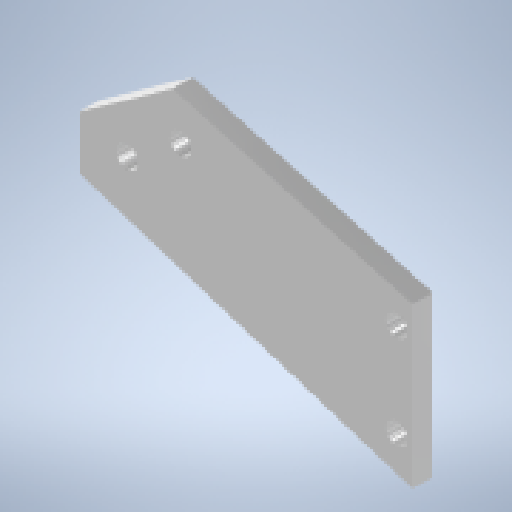
# Autodesk Inventor part: antana_side
Saved by Autodesk Inventor 2024.1 (Build 281209000, 209)
## iProperties
Created: 2024-02-25
Part Number: antana_side
Material: アルミニウム 6061
Document SubType Name: Sheet Metal
Designer: hibik
Density: 2.7 g/cm^3
Sheet Metal Rule: Default_mm
Appearance: アルミニウム - フラット
Author: hibik
Autodesk Inventor part; units mm, degrees
ref_plane "YZ Plane" through (0, 0, 0) normal (1, 0, 0) x (0, 1, 0)
ref_plane "XZ Plane" through (0, 0, 0) normal (0, 1, 0) x (-1, 0, 0)
ref_plane "XY Plane" through (0, 0, 0) normal (0, 0, 1) x (1, 0, 0)
sketch "スケッチ1" plane through (0, 0, 0) normal (0, 0, 1) x (1, 0, 0)
  line L0 (-25, 8) -> (-25, 12)
  line L1 (-25, 12) -> (0, 12)
  line L2 (0, 12) -> (0, 0)
  line L3 (0, 0) -> (-25, 8)
  line L4 (0, 12) -> (-18, 17)
  line L5 (-18, 17) -> (-25, 12)
  dimension "d0" = 12
  dimension "d2" = 4
  dimension "d4" = 25
  dimension "d7" = 5
  dimension "d8" = 18
  measures "d0" distance of L1.end L2.end
  measures "d2" distance of L0.start L0.end
  measures "d4" distance between parallel lines of L2 L0
  measures "d7" distance from line of L1 L4.end
  measures "d8" distance from line of L2 L4.end
extrude "プレート1" add sketch "スケッチ1" along normal blind 1.5
sketch "スケッチ4" plane through (0, 0, 0) normal (0, 0, -1) x (-1, 0, 0)
  circle A0 centre (1.5, 10) radius 0.8
  line L0 (0, 0) -> (0, 12) projected
  circle A1 centre (1.5, 3) radius 0.8
  circle A2 centre (14.9448, 13.0377) radius 0.8
  circle A3 centre (18.9448, 10.1806) radius 0.8
  line L1 (14.9448, 13.0377) -> (18.9448, 10.1806) construction
  line L2 (18, 17) -> (25, 12) projected
  line L3 (0, 12) -> (18, 17) projected
  dimension "d21" = 1.6
  dimension "d22" = 1.5
  dimension "d23" = 2
  dimension "d24" = 3
  dimension "d25" = 5
  dimension "d26" = 3
  dimension "d27" = 4
  constraints: 4 centre point, 3 equal radius, 2 end point, 1 parallel, 1 vertical alignment
  measures "d21" diameter of A0
  measures "d22" distance from line of L0 A0.centre
  measures "d23" vertical distance of L0.end A0.centre
  measures "d24" vertical distance of L0.start A1.centre
  measures "d25" distance between parallel lines of L2 L1
  measures "d26" distance from line of L3 L1.start
  measures "d27" horizontal distance of L1.start L1.end
extrude "切り取り1" cut sketch "スケッチ4" against normal blind 1.5
equation "\"d28\" = Thickness"
equation "\"d3\" = Thickness"
equation "\"BendRadius\" = Thickness"
equation "\"BendReliefWidth\" = Thickness"
equation "\"BendReliefDepth\" = 0.5 * Thickness"
equation "\"CornerReliefSize\" = 4 * Thickness"
equation "\"MinimumRemnant\" = 2 * Thickness"
equation "\"TransitionRadius\" = BendRadius"
equation "\"JacobiRadiusSize\" = BendRadius"
equation "\"GapSize\" = Thickness"
equation "\"Thickness\" = 1.5"
